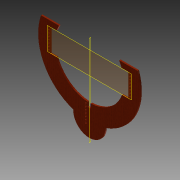
# Autodesk Inventor part: gyroYoke01
Saved by Autodesk Inventor 2013 (Build 170138000, 138)
## iProperties
Created: 2013-02-24
Part Number: gyroYoke01
Material: Wood (Oak)
Document SubType Name: Modeling
Designer: Nano
Density: 0.56 g/cm^3
Mass: 146.727 g
Surface Area: 937.732 cm^2
Volume: 262.012 cm^3
d0: 0.125 in
d1: 1.000 in
d3: 0.250 in
d4: 0.00 deg
d5: 0.250 in
d6: 0.250 in
d7: 0.250 in
d8: 0.250 in
d9: 0.125 in
d10: 0.125 in
d11: 0.250 in
d13: 0.250 in
d14: 0.00 deg
d15: 0.125 in
d22: 6.000 ul
d24: 0.500 in
d26: 0.00 deg
d12: 0.250 in
Author: Nano
Autodesk Inventor part; units mm, degrees
ref_plane "YZ Plane" through (0, 0, 0) normal (1, 0, 0) x (0, 1, 0)
ref_plane "XZ Plane" through (0, 0, 0) normal (0, 1, 0) x (-1, 0, 0)
ref_plane "XY Plane" through (0, 0, 0) normal (0, 0, 1) x (1, 0, 0)
ref_plane "Work Plane1" through (0, 0, 0) normal (0, 0, 1) x (1, 0, 0)
sketch "Sketch1" plane through (0, 0, 0) normal (0, 0, 1) x (1, 0, 0)
  circle A0 centre (166.6875, 44.45) radius 6.35 construction
  line L0 (0, 0) -> (333.375, 0) construction
  line L1 (333.375, 0) -> (333.375, 88.9) construction
  line L2 (0, 88.9) -> (333.375, 88.9) construction
  line L3 (0, 0) -> (0, 88.9) construction
  line L4 (336.55, 95.25) -> (336.55, -6.35)
  line L5 (-3.175, -6.35) -> (-3.175, 95.25)
  arc A1 (374.8561, -33.4017) -> (376.2621, 118.4333) centre (166.6875, 44.45) ccw
  arc A2 (97.9077, -166.8895) -> (235.4673, -166.8895) centre (166.6875, -179.07) ccw
  arc A3 (235.4673, -166.8895) -> (236.492, -166.5533) centre (166.6875, 44.45) ccw
  arc A4 (-41.4811, -33.4017) -> (96.883, -166.5533) centre (166.6875, 44.45) ccw
  arc A5 (-43.1277, 117.7484) -> (-41.4811, -33.4017) centre (166.6875, 44.45) ccw
  arc A6 (336.55, 165.3087) -> (333.375, 169.6513) centre (166.6875, 44.45) ccw
  arc A7 (0, 169.6513) -> (-3.175, 165.3087) centre (166.6875, 44.45) ccw
  line L6 (376.2621, 118.4333) -> (296.5092, 118.3031)
  line L7 (35.5855, 117.8769) -> (-43.1277, 117.7484)
  arc A8 (194.8672, -103.8723) -> (308.8598, -6.35) centre (166.6875, 44.45) ccw
  arc A9 (307.1415, 95.25) -> (296.5092, 118.3031) centre (166.6875, 44.45) ccw
  arc A10 (35.5855, 117.8769) -> (25.271, 95.25) centre (166.6875, 44.45) ccw
  arc A11 (24.5152, -6.35) -> (136.5493, -103.4867) centre (166.6875, 44.45) ccw
  line L8 (-3.175, 95.25) -> (25.271, 95.25)
  line L9 (307.1415, 95.25) -> (336.55, 95.25)
  line L10 (336.55, -6.35) -> (308.8598, -6.35)
  line L11 (24.5152, -6.35) -> (-3.175, -6.35)
  line L12 (173.0375, -106.3919) -> (173.0375, -125.2673)
  line L13 (173.0375, -125.2673) -> (160.3375, -125.2673)
  line L14 (160.3375, -125.2673) -> (160.3375, -106.3919)
  line L15 (163.5125, -117.9837) -> (169.8625, -117.9837) projected
  line L16 (166.6875, 44.45) -> (38.9307, -83.3068) projected
  arc A12 (136.5493, -103.4867) -> (160.3375, -106.3919) centre (166.6875, 44.45) ccw
  arc A13 (173.0375, -106.3919) -> (194.8672, -103.8723) centre (166.6875, 44.45) ccw
  arc A14 (236.492, -166.5533) -> (96.883, -166.5533) centre (166.6875, -169.0753) ccw
  arc A15 (236.492, -166.5533) -> (374.8561, -33.4017) centre (166.6875, 44.45) ccw
  arc A16 (96.883, -166.5533) -> (97.9077, -166.8895) centre (166.6875, 44.45) ccw
  arc A17 (96.883, -166.5533) -> (236.492, -166.5533) centre (166.6875, -169.0753) ccw
  point P0 (166.6875, -117.9837)
  dimension "d0" = 3.175
  dimension "d5" = 6.35
  dimension "d6" = 6.35
  dimension "d7" = 6.35
  dimension "d8" = 6.35
  dimension "d9" = 3.175
  dimension "d10" = 3.175
  dimension "d11" = 6.35
  dimension "d12" = 6.35
  dimension "d47" = 139.7
  dimension "d58" = 223.52
  dimension "d59" = 69.85
  dimension "d60" = 222.25
  dimension "d61" = 222.25
  dimension "d62" = 222.25
  dimension "d63" = 222.25
  constraints: 34 point on circle, 22 end point, 17 centre point, 4 point on line, 2 vertical alignment, 1 coincident, 1 collinear, 1 parallel, 1 other
  measures "d0" distance between parallel lines of L4 L1
  measures "d5" distance between parallel lines of L2 L9
  measures "d6" distance between parallel lines of L0 L10
  measures "d7" distance between parallel lines of L2 L8
  measures "d8" distance between parallel lines of L0 L11
  measures "d9" distance from line of L14 L15.start
  measures "d10" distance from line of L15.end L12
  measures "d11" distance from line of L12 point (166.688, -117.984)
  measures "d12" distance from line of point (166.688, -117.984) L14
  measures "d47" diameter of A14
  measures "d58" distance of A2.centre L16.start
  measures "d59" radius of A2
  measures "d60" radius of A15
  measures "d61" radius of A4
  measures "d62" radius of A1
  measures "d63" radius of A5
extrude "Extrusion1" add sketch "Sketch1" against normal blind 6.35 contours L9 A9 L6 A1 A15 A14 A13 A8 L10 L4 | A14 A3 A2 A17 A16 A12 L14 L13 L12 A13 | A17 A2 A3 | A14 A4 A5 L7 A10 L8 L5 L11 A11 A12 | A16 A2 A17
sketch "Sketch2" plane through (0, 0, 0) normal (0, 0, 1) x (1, 0, 0)
  line L0 (339.725, 79.375) -> (346.075, 79.375) projected
  line L1 (346.075, 85.725) -> (346.075, 79.375) projected
  line L2 (346.075, 85.725) -> (339.725, 85.725) projected
  line L3 (339.725, 85.725) -> (339.725, 79.375) projected
  line L4 (339.725, 66.675) -> (346.075, 66.675) projected
  line L5 (346.075, 73.025) -> (346.075, 66.675) projected
  line L6 (346.075, 73.025) -> (339.725, 73.025) projected
  line L7 (339.725, 73.025) -> (339.725, 66.675) projected
  line L8 (339.725, 53.975) -> (346.075, 53.975) projected
  line L9 (346.075, 60.325) -> (346.075, 53.975) projected
  line L10 (346.075, 60.325) -> (339.725, 60.325) projected
  line L11 (339.725, 60.325) -> (339.725, 53.975) projected
  line L12 (346.075, 47.625) -> (339.725, 47.625) projected
  line L13 (339.725, 47.625) -> (339.725, 41.275) projected
  line L14 (339.725, 41.275) -> (346.075, 41.275) projected
  line L15 (346.075, 47.625) -> (346.075, 41.275) projected
  line L16 (346.075, 34.925) -> (339.725, 34.925) projected
  line L17 (339.725, 34.925) -> (339.725, 28.575) projected
  line L18 (339.725, 28.575) -> (346.075, 28.575) projected
  line L19 (346.075, 34.925) -> (346.075, 28.575) projected
  line L20 (346.075, 22.225) -> (339.725, 22.225) projected
  line L21 (339.725, 22.225) -> (339.725, 15.875) projected
  line L22 (339.725, 15.875) -> (346.075, 15.875) projected
  line L23 (346.075, 22.225) -> (346.075, 15.875) projected
  line L24 (346.075, 9.525) -> (339.725, 9.525) projected
  line L25 (339.725, 9.525) -> (339.725, 3.175) projected
  line L26 (339.725, 3.175) -> (346.075, 3.175) projected
  line L27 (346.075, 9.525) -> (346.075, 3.175) projected
  point P0 (0, 0)
extrude "Extrusion2" cut sketch "Sketch2" against normal blind 6.35
sketch "Sketch3" plane through (0, 0, 0) normal (0, 0, 1) x (1, 0, 0)
  line L0 (339.725, 15.875) -> (346.075, 9.525) construction
  line L1 (346.075, 15.875) -> (339.725, 9.525) construction
  point P0 (0, 0)
  point P1 (342.9, 12.7)
  constraints: 4 end point
hole "Hole1" at (342.9, 12.7, 0) direction (0, 0, -1) diameter 3.175 end through all
pattern_linear "Rectangular Pattern1" count 6 spacing 12.7 along (0, 1, 0) of "Hole1"
sketch "Sketch5" plane through (0, 0, 0) normal (0, 0, 1) x (1, 0, 0)
  line L0 (147.6375, -110.6581) -> (147.6375, -116.7384)
  line L1 (153.9875, -110.6581) -> (153.9875, -116.7384)
  line L2 (153.9875, -110.6581) -> (153.9875, -116.7384)
  line L3 (147.6375, -110.6581) -> (147.6375, -116.7384)
  line L4 (147.6375, -110.6581) -> (147.6375, -116.7384)
  line L5 (153.9875, -110.6581) -> (153.9875, -116.7384)
  line L6 (153.9875, -110.6581) -> (153.9875, -116.7384)
  line L7 (147.6375, -110.6581) -> (147.6375, -116.7384)
  line L8 (147.6375, -110.6581) -> (147.6375, -116.7384)
  line L9 (153.9875, -110.6581) -> (153.9875, -116.7384)
  line L10 (153.9875, -110.6581) -> (153.9875, -116.7384)
  line L11 (147.6375, -110.6581) -> (147.6375, -116.7384)
  line L12 (147.6375, -110.6581) -> (147.6375, -116.7384)
  line L13 (153.9875, -110.6581) -> (153.9875, -116.7384)
  line L14 (147.6375, -116.7384) -> (153.9875, -116.7384)
  line L15 (153.9875, -110.6581) -> (147.6375, -110.6581)
  line L16 (147.6375, -116.7384) -> (153.9875, -116.7384)
  line L17 (153.9875, -110.6581) -> (147.6375, -110.6581)
  line L18 (147.6375, -116.7384) -> (153.9875, -116.7384)
  line L19 (153.9875, -110.6581) -> (147.6375, -110.6581)
  line L20 (147.6375, -116.7384) -> (153.9875, -116.7384)
  line L21 (153.9875, -110.6581) -> (147.6375, -110.6581)
  line L22 (147.6375, -116.7384) -> (153.9875, -116.7384)
  line L23 (153.9875, -110.6581) -> (147.6375, -110.6581)
  line L24 (147.6375, -116.7384) -> (153.9875, -116.7384)
  line L25 (153.9875, -110.6581) -> (147.6375, -110.6581)
  line L26 (147.6375, -116.7384) -> (153.9875, -116.7384)
  line L27 (153.9875, -110.6581) -> (147.6375, -110.6581)
  line L28 (147.6375, -123.0884) -> (153.9875, -123.0884) projected
  line L29 (147.6375, -123.0884) -> (147.6375, -129.4384) projected
  line L30 (153.9875, -129.4384) -> (147.6375, -129.4384) projected
  line L31 (153.9875, -142.1384) -> (147.6375, -142.1384) projected
  line L32 (147.6375, -135.7884) -> (153.9875, -135.7884) projected
  line L33 (147.6375, -135.7884) -> (147.6375, -142.1384) projected
  line L34 (147.6375, -148.4884) -> (153.9875, -148.4884) projected
  line L35 (147.6375, -148.4884) -> (147.6375, -154.8384) projected
  line L36 (153.9875, -154.8384) -> (147.6375, -154.8384) projected
  line L37 (153.9875, -167.5384) -> (147.6375, -167.5384) projected
  line L38 (147.6375, -161.1884) -> (153.9875, -161.1884) projected
  line L39 (147.6375, -161.1884) -> (147.6375, -167.5384) projected
  line L40 (147.6375, -173.8884) -> (153.9875, -173.8884) projected
  line L41 (147.6375, -173.8884) -> (147.6375, -180.2384) projected
  line L42 (153.9875, -180.2384) -> (147.6375, -180.2384) projected
  line L43 (147.6375, -110.6581) -> (147.6375, -116.7384) projected
  line L44 (153.9875, -116.7384) -> (147.6375, -116.7384) projected
  line L45 (153.9875, -110.6581) -> (153.9875, -116.7384) projected
  line L46 (153.9875, -110.6581) -> (147.6375, -110.6581) projected
  line L47 (153.9875, -173.8884) -> (153.9875, -180.2384) projected
  line L48 (153.9875, -161.1884) -> (153.9875, -167.5384) projected
  line L49 (153.9875, -148.4884) -> (153.9875, -154.8384) projected
  line L50 (153.9875, -135.7884) -> (153.9875, -142.1384) projected
  line L51 (153.9875, -123.0884) -> (153.9875, -129.4384) projected
  line L52 (147.6375, -186.5884) -> (153.9875, -186.5884) projected
  line L53 (147.6375, -186.5884) -> (147.6375, -192.9384) projected
  line L54 (153.9875, -192.9384) -> (147.6375, -192.9384) projected
  line L55 (153.9875, -186.5884) -> (153.9875, -192.9384) projected
  point P0 (0, 0)
  constraints: 56 end point
extrude "Extrusion3" cut sketch "Sketch5" against normal through all
sketch "Sketch6" plane through (0, 0, 0) normal (0, 0, 1) x (1, 0, 0)
  circle A0 centre (342.9, 76.2) radius 1.5875 construction
  circle A1 centre (342.9, 63.5) radius 1.5875 construction
  circle A2 centre (342.9, 50.8) radius 1.5875 construction
  circle A3 centre (342.9, 38.1) radius 1.5875 construction
  circle A4 centre (342.9, 25.4) radius 1.5875 construction
  circle A5 centre (342.9, 12.7) radius 1.5875 construction
  line L0 (339.725, 15.875) -> (339.725, 22.225) construction
  line L1 (339.725, 22.225) -> (346.075, 22.225) construction
  line L2 (346.075, 22.225) -> (346.075, 15.875) construction
  line L3 (346.075, 15.875) -> (339.725, 15.875) construction
  line L4 (339.725, 41.275) -> (339.725, 47.625) construction
  line L5 (339.725, 47.625) -> (346.075, 47.625) construction
  line L6 (346.075, 47.625) -> (346.075, 41.275) construction
  line L7 (346.075, 41.275) -> (339.725, 41.275) construction
  line L8 (346.075, 73.025) -> (346.075, 66.675) construction
  line L9 (346.075, 66.675) -> (339.725, 66.675) construction
  line L10 (339.725, 66.675) -> (339.725, 73.025) construction
  line L11 (339.725, 73.025) -> (346.075, 73.025) construction
  line L12 (346.075, 85.725) -> (346.075, 79.375) construction
  line L13 (346.075, 79.375) -> (339.725, 79.375) construction
  line L14 (339.725, 79.375) -> (339.725, 85.725) construction
  line L15 (339.725, 85.725) -> (346.075, 85.725) construction
  line L16 (346.075, 60.325) -> (346.075, 53.975) construction
  line L17 (346.075, 53.975) -> (339.725, 53.975) construction
  line L18 (339.725, 53.975) -> (339.725, 60.325) construction
  line L19 (339.725, 60.325) -> (346.075, 60.325) construction
  line L20 (339.725, 28.575) -> (339.725, 34.925) construction
  line L21 (339.725, 34.925) -> (346.075, 34.925) construction
  line L22 (346.075, 34.925) -> (346.075, 28.575) construction
  line L23 (346.075, 28.575) -> (339.725, 28.575) construction
  line L24 (339.725, 3.175) -> (339.725, 9.525) construction
  line L25 (339.725, 9.525) -> (346.075, 9.525) construction
  line L26 (346.075, 9.525) -> (346.075, 3.175) construction
  line L27 (346.075, 3.175) -> (339.725, 3.175) construction
  line L28 (336.55, 95.25) -> (336.55, -6.35) construction
  line L29 (336.55, -6.35) -> (308.8598, -6.35) construction
  arc A6 (173.0375, -106.3919) -> (308.8598, -6.35) centre (166.6875, 44.45) ccw construction
  arc A7 (24.5152, -6.35) -> (160.3375, -106.3919) centre (166.6875, 44.45) ccw construction
  line L30 (24.5152, -6.35) -> (-3.175, -6.35) construction
  line L31 (-3.175, -6.35) -> (-3.175, 95.25) construction
  line L32 (-3.175, 95.25) -> (25.271, 95.25) construction
  arc A8 (35.5855, 117.8769) -> (25.271, 95.25) centre (166.6875, 44.45) ccw construction
  line L33 (35.5855, 117.8769) -> (-43.1277, 117.7484) construction
  arc A9 (-43.1277, 117.7484) -> (96.883, -166.5533) centre (166.6875, 44.45) ccw construction
  arc A10 (236.492, -166.5533) -> (376.2621, 118.4333) centre (166.6875, 44.45) ccw construction
  line L34 (376.2621, 118.4333) -> (296.5092, 118.3031) construction
  arc A11 (307.1415, 95.25) -> (296.5092, 118.3031) centre (166.6875, 44.45) ccw construction
  line L35 (307.1415, 95.25) -> (336.55, 95.25) construction
  line L36 (147.6375, -180.2384) -> (153.9875, -186.5884) construction
  line L37 (153.9875, -180.2384) -> (147.6375, -186.5884) construction
  arc A12 (96.883, -166.5533) -> (236.492, -166.5533) centre (166.6875, -169.0753) ccw projected
  line L38 (173.0375, -106.3919) -> (173.0375, -125.2673) projected
  line L39 (173.0375, -125.2673) -> (160.3375, -125.2673) projected
  line L40 (160.3375, -125.2673) -> (160.3375, -106.3919) projected
  point P0 (0, 0)
  point P1 (150.8125, -183.4134)
  constraints: 4 end point
hole "Hole4" at (150.8125, -183.4134, 0) direction (0, 0, -1) diameter 3.175 end through all
pattern_linear "Rectangular Pattern4" count 6 spacing 12.7 along (0, 1, 0) of "Hole4"
ref_plane "Work Plane3" through (166.6875, -125.2673, -119.0625) normal (-1, 0, 0) x (0, 0, 1)
ref_plane "Work Plane5" through (166.6875, -178.3136, -60.56) normal (-1, 0, 0) x (0, 0, -1)
mirror "Mirror4" about plane through (166.6875, -178.3136, -60.56) normal (-1, 0, 0) of "Extrusion2", "Hole1", "Rectangular Pattern1"
equation "\"d6\" = d5"
equation "\"d7\" = d5"
equation "\"d8\" = d5"
equation "\"d10\" = d9"
body "Solid1"
